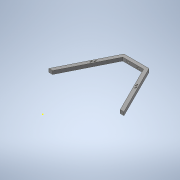
# Autodesk Inventor part: Cavalete_Inferior
Saved by Autodesk Inventor 2022 (Build 260153000, 153)
## iProperties
Manager: Standard
Created: 2016-02-21
Part Number: Cavalete_Inferior
Material: SAE 1010/1020
Document SubType Name: Modeling
Designer: Everton
Authority: Rafael Salvador
Manufacturer: Standard
Standards Organization: Custom
Density: 7.86 g/cm^3
Appearance: Steel
Mass: 19558.2 g
Surface Area: 2597.77 cm^2
Volume: 2488.33 cm^3
Author: Everton
Comments: -
Revision Number: 00
Autodesk Inventor part; units mm, degrees
ref_plane "YZ Plane" through (0, 0, 0) normal (1, 0, 0) x (0, 1, 0)
ref_plane "XZ Plane" through (0, 0, 0) normal (0, 1, 0) x (-1, 0, 0)
ref_plane "XY Plane" through (0, 0, 0) normal (0, 0, 1) x (1, 0, 0)
sketch "Sketch1" plane through (0, 0, 0) normal (0, 0, 1) x (1, 0, 0)
  line L0 (9.7407, 1114.2593) -> (159.7407, 1114.2593)
  line L1 (9.7407, 1114.2593) -> (-140.2593, 1114.2593)
  line L2 (-290.2593, 814.2593) -> (-140.2593, 1114.2593)
  line L3 (159.7407, 1114.2593) -> (459.7407, 514.2593)
  line L4 (135.0194, 1074.2593) -> (9.7407, 1074.2593)
  line L5 (9.7407, 1074.2593) -> (-115.5379, 1074.2593)
  line L6 (-115.5379, 1074.2593) -> (-245.5379, 814.2593)
  line L7 (9.7407, 1114.2593) -> (159.7407, 1114.2593)
  line L8 (9.7407, 1114.2593) -> (-140.2593, 1114.2593)
  line L9 (-440.2593, 514.2593) -> (-140.2593, 1114.2593)
  line L10 (159.7407, 1114.2593) -> (309.9483, 813.8441)
  line L11 (135.0194, 1074.2593) -> (9.7407, 1074.2593)
  line L12 (9.7407, 1074.2593) -> (-115.5379, 1074.2593)
  line L13 (-115.5379, 1074.2593) -> (-245.5379, 814.2593)
  line L14 (-245.5379, 814.2593) -> (-290.2593, 814.2593)
  line L15 (265.227, 813.8441) -> (309.9483, 813.8441)
  line L16 (265.227, 813.8441) -> (135.0194, 1074.2593)
  line L17 (415.0194, 514.2593) -> (135.0194, 1074.2593)
  line L18 (-395.5379, 514.2593) -> (-440.2593, 514.2593)
  line L19 (-245.5379, 814.2593) -> (-395.5379, 514.2593)
  line L20 (-440.2593, 514.2593) -> (-395.5379, 514.2593)
  line L21 (415.0194, 514.2593) -> (459.7407, 514.2593)
  point P0 (0, 0)
  dimension "d13" = 300
  constraints: 44 end point, 4 horizontal, 2 point on line, 1 midpoint
  measures "d13" distance from line of L6.end L1
extrude "Extrusion1" add sketch "Sketch1" along normal blind 40 contours L0 L3 L15 L16 L4 L5 L6 L14 L2 L1
fillet "Fillet2" radius 0.5 1 edges at (200.1232, 944.0517, 0)
fillet "Fillet3" radius 0.5 3 edges at (159.7407, 1114.2593, 20) (84.7407, 1114.2593, 0) (-215.2593, 964.2593, 0)
sketch "Sketch2" plane through (-140.2593, 1114.2593, 0.5) normal (0, 1, 0) x (1, 0, 0)
  line L0 (300.1382, -39.5) -> (300.1382, 0.4472) projected
  line L1 (300.1382, -19.5) -> (0, -19.5)
  line L2 (0, 0) -> (0, -39.5) projected
  circle A0 centre (150.0691, -19.5) radius 1.5
  point P0 (140.2593, 0.5)
  point P1 (300.1382, -39)
  point P2 (300.1382, 0)
  point P3 (0, -39)
  dimension "d14" = 3
  constraints: 2 end point, 2 point on line, 1 centre point, 1 midpoint
  measures "d14" diameter of A0
extrude "Extrusion2" cut sketch "Sketch2" against normal blind 10
extrude "Extrusion3" add sketch "Sketch1" along normal blind 40 contours L3 L21 L17 L15 | L14 L19 L18 L9
sketch "Sketch3" plane through (-140.2593, 1114.2593, 0.5) normal (0, 1, 0) x (1, 0, 0)
  point P0 (140.2593, 0.5)
sketch "Sketch4" plane through (-140.2593, 1114.2593, 0.5) normal (0, 1, 0) x (1, 0, 0)
  circle A0 centre (150.0691, -19.5) radius 1.5 projected
  line L0 (0, 0) -> (299.691, 0) projected
  line L1 (0, 0) -> (0, -39.5) projected
  line L2 (299.691, 0) -> (299.691, -39.5) projected
  line L3 (200.1691, -14.5) -> (225.9691, -14.5) projected
  line L4 (225.9691, -24.5) -> (200.1691, -24.5) projected
  arc A1 (225.9691, -24.5) -> (225.9691, -14.5) centre (225.9691, -19.5) ccw projected
  arc A2 (200.1691, -14.5) -> (200.1691, -24.5) centre (200.1691, -19.5) ccw projected
  arc A3 (74.1691, -14.5) -> (74.1691, -24.5) centre (74.1691, -19.5) ccw projected
  line L5 (74.1691, -14.5) -> (99.9691, -14.5) projected
  line L6 (74.1691, -24.5) -> (99.9691, -24.5) projected
  arc A4 (99.9691, -24.5) -> (99.9691, -14.5) centre (99.9691, -19.5) ccw projected
  line L7 (299.691, -39.5) -> (0, -39.5) projected
  point P0 (140.2593, 0.5)
extrude "Extrusion4" cut sketch "Sketch4" against normal blind 50 contours L3 A1 L4 A2 | L5 A4 L6 A3
sketch "Esboço5" plane through (0, 0, 0) normal (0, 0, 1) x (1, 0, 0)
  line L0 (159.4317, 1114.2593) -> (-140.2593, 1114.2593) projected
  line L1 (-94.9789, 1114.2593) -> (-94.9789, 897.5465)
  line L2 (-94.9789, 897.5465) -> (-260.935, 897.5465)
  line L3 (-290.2593, 814.2593) -> (-140.2593, 1114.2593) projected
  line L4 (-250.2227, 877.5465) -> (-250.2227, 857.5465)
  line L5 (265.227, 813.8441) -> (135.0194, 1074.2593) projected
  line L6 (223.3758, 897.5465) -> (233.3758, 897.5465)
  line L7 (233.3758, 897.5465) -> (233.3758, 882.5465)
  line L8 (-94.9789, 897.5465) -> (445.9224, 897.5465)
  line L9 (268.1798, 897.5465) -> (258.1798, 897.5465)
  line L10 (268.1798, 897.5465) -> (258.1798, 897.5465)
  line L11 (258.1798, 897.5465) -> (258.1798, 882.5465)
  line L12 (258.1798, 882.5465) -> (258.1798, 877.5465)
  line L13 (258.1798, 862.5465) -> (258.1798, 857.5465)
  line L14 (258.1798, 857.5465) -> (258.1798, 852.5465)
  arc A0 (253.1798, 857.5465) -> (263.1798, 857.5465) centre (258.1798, 857.5465) ccw
  arc A1 (263.1798, 877.5465) -> (253.1798, 877.5465) centre (258.1798, 877.5465) ccw
  line L15 (263.1798, 877.5465) -> (263.1798, 857.5465)
  line L16 (253.1798, 857.5465) -> (253.1798, 877.5465)
  line L17 (-248.6157, 897.5465) -> (-293.337, 808.1037)
  line L18 (268.1798, 897.5465) -> (312.835, 808.0707)
  line L19 (459.7407, 514.2593) -> (159.9907, 1113.7593) projected
  line L20 (-293.337, 808.1037) -> (-248.6157, 808.1037)
  line L21 (-395.5379, 514.2593) -> (-115.5379, 1074.2593) projected
  line L22 (-248.6157, 808.1037) -> (-258.6157, 808.1037)
  line L23 (-258.6157, 808.1037) -> (-258.6157, 823.1037)
  line L24 (-258.6157, 823.1037) -> (-258.6157, 828.1037)
  line L25 (-258.6157, 848.1037) -> (-258.6157, 853.1037)
  arc A2 (-253.6157, 848.1037) -> (-263.6157, 848.1037) centre (-258.6157, 848.1037) ccw
  arc A3 (-263.6157, 828.1037) -> (-253.6157, 828.1037) centre (-258.6157, 828.1037) ccw
  line L26 (-263.6157, 828.1037) -> (-263.6157, 848.1037)
  line L27 (-253.6157, 848.1037) -> (-253.6157, 828.1037)
  line L28 (-258.6157, 828.1037) -> (-258.6157, 833.1037)
  line L29 (-258.6157, 843.1037) -> (-258.6157, 848.1037)
  line L30 (312.835, 808.0707) -> (268.1137, 808.0707)
  line L31 (135.0194, 1074.2593) -> (415.0194, 514.2593) projected
  line L32 (268.1137, 808.0707) -> (278.1137, 808.0707)
  line L33 (278.1137, 808.0707) -> (278.1137, 823.0707)
  line L34 (278.1137, 823.0707) -> (278.1137, 828.0707)
  line L35 (278.1137, 848.0707) -> (278.1137, 853.0707)
  arc A4 (283.1137, 848.0707) -> (273.1137, 848.0707) centre (278.1137, 848.0707) ccw
  arc A5 (273.1137, 828.0707) -> (283.1137, 828.0707) centre (278.1137, 828.0707) ccw
  line L36 (273.1137, 848.0707) -> (273.1137, 828.0707)
  line L37 (283.1137, 848.0707) -> (283.1137, 828.0707)
  line L38 (278.1137, 828.0707) -> (278.1137, 833.0707)
  line L39 (278.1137, 843.0707) -> (278.1137, 848.0707)
  line L40 (-238.6157, 882.5465) -> (-238.6157, 862.5465)
  line L41 (-233.6157, 862.5465) -> (-233.6157, 882.5465)
  line L42 (-243.6157, 882.5465) -> (-243.6157, 862.5465)
  line L43 (-248.6157, 897.5465) -> (-238.6157, 897.5465)
  line L44 (-238.6157, 897.5465) -> (-238.6157, 882.5465)
  line L45 (-293.337, 808.1037) -> (-248.6157, 808.1037)
  line L46 (-248.6157, 897.5465) -> (-238.6157, 897.5465)
  line L47 (-238.6157, 897.5465) -> (-238.6157, 882.5465)
  line L48 (-238.6157, 882.5465) -> (-238.6157, 877.5465)
  line L49 (-238.6157, 857.5465) -> (-238.6157, 852.5465)
  arc A6 (-243.6157, 857.5465) -> (-233.6157, 857.5465) centre (-238.6157, 857.5465) ccw
  arc A7 (-233.6157, 877.5465) -> (-243.6157, 877.5465) centre (-238.6157, 877.5465) ccw
  line L50 (-243.6157, 877.5465) -> (-243.6157, 857.5465)
  line L51 (-233.6157, 857.5465) -> (-233.6157, 877.5465)
  line L52 (-238.6157, 877.5465) -> (-238.6157, 872.5465)
  line L53 (-238.6157, 862.5465) -> (-238.6157, 857.5465)
  point P0 (0, 0)
  dimension "d23" = 216.7128
  dimension "d33" = 10
  dimension "d34" = 15
  dimension "d35" = 5
  dimension "d37" = 20
  dimension "d38" = 5
  dimension "d39" = 10
  dimension "d40" = 100
  dimension "d41" = 100
  dimension "d42" = 10
  dimension "d43" = 15
  dimension "d44" = 5
  dimension "d45" = 20
  dimension "d46" = 5
  dimension "d47" = 10
  dimension "d48" = 10
  dimension "d49" = 10
  dimension "d50" = 15
  dimension "d51" = 5
  dimension "d52" = 20
  dimension "d53" = 5
  dimension "d54" = 10
  dimension "d55" = 10
  dimension "d69" = 10
  dimension "d70" = 15
  dimension "d71" = 5
  dimension "d72" = 20
  dimension "d73" = 5
  dimension "d74" = 10
  dimension "d75" = 10
  constraints: 96 end point, 21 point on line, 18 point on circle, 9 coincident, 8 centre point, 7 tangent, 6 perpendicular, 4 collinear, 4 horizontal, 2 vertical, 1 parallel
  measures "d23" distance of L1.start L1.end
  measures "d33" distance of L9.start L9.end
  measures "d34" distance of L9.end L11.end
  measures "d35" distance of L11.end L12.end
  measures "d37" distance of L12.end L13.end
  measures "d38" distance of L13.end L14.end
  measures "d39" diameter of A1
  measures "d40" distance of L17.start L17.end
  measures "d41" distance of L9.start L18.end
  measures "d42" distance of L20.end L22.end
  measures "d43" distance of L22.end L23.end
  measures "d44" distance of L23.end L24.end
  measures "d45" distance of L24.end L25.start
  measures "d46" distance of L25.start L25.end
  measures "d47" diameter of A2
  measures "d48" diameter of A3
  measures "d49" distance of L30.end L32.end
  measures "d50" distance of L32.end L33.end
  measures "d51" distance of L33.end L34.end
  measures "d52" distance of L34.end L35.start
  measures "d53" distance of L35.start L35.end
  measures "d54" diameter of A4
  measures "d55" diameter of A5
  measures "d69" distance of L17.start L43.end
  measures "d70" distance of L43.end L44.end
  measures "d71" distance of L44.end L48.end
  measures "d72" distance of L48.end L49.start
  measures "d73" distance of L49.start L49.end
  measures "d74" diameter of A6
  measures "d75" diameter of A7
extrude "Extrusão5" cut sketch "Esboço5" along normal mid plane 1000 contours A5 L36 A4 L37 | A1 L15 A0 L16 | A3 L26 A2 L27 | A7 L41 L51 A6 L49 L53 L40 | L40 L53 L49 A6 L50 L42 A7
sketch "Esboço8" plane through (0, 0, 40) normal (0, 0, 1) x (1, 0, 0)
  point P0 (0, 0)
body "Solid1"
